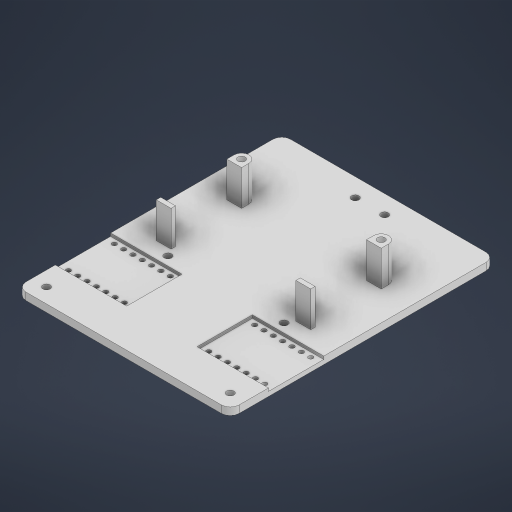
# Autodesk Inventor part: chasis
Saved by Autodesk Inventor 2023 (Build 270158000, 158)
## iProperties
Created: 2022-08-21
Part Number: chasis
Material: Generic
Document SubType Name: Modeling
Designer: marat
Density: 1 g/cm^3
Appearance: Default
Author: marat
Autodesk Inventor part; units mm, degrees
ref_plane "YZ Plane" through (0, 0, 0) normal (1, 0, 0) x (0, 1, 0)
ref_plane "XZ Plane" through (0, 0, 0) normal (0, 1, 0) x (-1, 0, 0)
ref_plane "XY Plane" through (0, 0, 0) normal (0, 0, 1) x (1, 0, 0)
sketch "Sketch3" plane through (0, 0, 0) normal (0, 1, 0) x (-1, 0, 0)
  line L0 (72.5, 90) -> (-72.5, 90)
  line L1 (-72.5, 90) -> (-72.5, -90)
  line L2 (-72.5, -90) -> (72.5, -90)
  line L3 (72.5, -90) -> (72.5, 90)
  line L4 (72.5, 90) -> (-72.5, -90) construction
  line L5 (-72.5, 90) -> (72.5, -90) construction
  point P0 (0, 0)
  dimension "d7" = 145
  dimension "d8" = 180
  constraints: 12 end point, 2 midpoint, 2 parallel, 1 horizontal, 1 perpendicular
  measures "d7" distance of L2.end L1.end
  measures "d8" distance of L1.end L0.end
extrude "Extrusion3" add sketch "Sketch3" along normal blind 5
sketch "Sketch4" plane through (0, 5, 0) normal (0, 1, 0) x (1, 0, 0)
  line L0 (23.935, -64) -> (72.5, -64)
  line L1 (72.5, -64) -> (72.5, -26.408)
  line L2 (72.5, -26.408) -> (23.935, -26.408)
  line L3 (23.935, -26.408) -> (23.935, -64)
  line L4 (23.935, -64) -> (72.5, -26.408) construction
  line L5 (72.5, -64) -> (23.935, -26.408) construction
  line L6 (72.5, -90) -> (72.5, 90) projected
  line L7 (-72.5, -90) -> (72.5, -90) projected
  line L8 (-72.5, -64) -> (-23.935, -64)
  line L9 (-23.935, -64) -> (-23.935, -26.408)
  line L10 (-23.935, -26.408) -> (-72.5, -26.408)
  line L11 (-72.5, -26.408) -> (-72.5, -64)
  line L12 (-72.5, -64) -> (-23.935, -26.408) construction
  line L13 (-23.935, -64) -> (-72.5, -26.408) construction
  line L14 (-72.5, 90) -> (-72.5, -90) projected
  point P0 (0, 0)
  point P1 (48.2175, -45.204)
  point P2 (-48.2175, -45.204)
  dimension "d11" = 48.565
  dimension "d12" = 37.592
  dimension "d13" = 0
  dimension "d14" = 26
  dimension "d20" = 48.565
  dimension "d21" = 37.592
  dimension "d22" = 0
  dimension "d23" = 26
  constraints: 24 end point, 4 midpoint, 4 parallel, 2 horizontal, 2 perpendicular
  measures "d11" distance of L2.end L1.end
  measures "d12" distance of L1.end L0.end
  measures "d13" distance between parallel lines of L6 L1
  measures "d14" distance between parallel lines of L7 L0
  measures "d20" distance of L10.end L9.end
  measures "d21" distance of L9.end L8.end
  measures "d22" distance between parallel lines of L14 L11
  measures "d23" distance between parallel lines of L7 L8
extrude "Extrusion4" cut sketch "Sketch4" against normal blind 2
sketch "Sketch5" plane through (0, 3, 0) normal (0, 1, 0) x (1, 0, 0)
  circle A0 centre (66.797, -60.825) radius 1.588
  line L0 (72.5, -26.408) -> (72.5, -64)
  line L1 (72.5, -64) -> (23.935, -64)
  circle A1 centre (60.447, -60.825) radius 1.588
  circle A2 centre (54.097, -60.825) radius 1.588
  circle A3 centre (47.747, -60.825) radius 1.588
  circle A4 centre (41.397, -60.825) radius 1.588
  circle A5 centre (35.047, -60.825) radius 1.588
  circle A6 centre (28.697, -60.825) radius 1.588
  circle A7 centre (66.797, -29.583) radius 1.588
  circle A8 centre (60.447, -29.583) radius 1.588
  circle A9 centre (54.097, -29.583) radius 1.588
  circle A10 centre (47.747, -29.583) radius 1.588
  circle A11 centre (41.397, -29.583) radius 1.588
  circle A12 centre (35.047, -29.583) radius 1.588
  circle A13 centre (28.697, -29.583) radius 1.588
  circle A14 centre (-66.797, -60.825) radius 1.588
  line L2 (-23.935, -64) -> (-72.5, -64) projected
  line L3 (-72.5, -64) -> (-72.5, -26.408) projected
  circle A15 centre (-60.447, -60.825) radius 1.588
  circle A16 centre (-54.097, -60.825) radius 1.588
  circle A17 centre (-47.747, -60.825) radius 1.588
  circle A18 centre (-41.397, -60.825) radius 1.588
  circle A19 centre (-35.047, -60.825) radius 1.588
  circle A20 centre (-28.697, -60.825) radius 1.588
  circle A21 centre (-66.797, -29.583) radius 1.588
  circle A22 centre (-60.447, -29.583) radius 1.588
  circle A23 centre (-54.097, -29.583) radius 1.588
  circle A24 centre (-47.747, -29.583) radius 1.588
  circle A25 centre (-41.397, -29.583) radius 1.588
  circle A26 centre (-35.047, -29.583) radius 1.588
  circle A27 centre (-28.697, -29.583) radius 1.588
  point P0 (0, 0)
  dimension "d24" = 3.176
  dimension "d25" = 5.703
  dimension "d26" = 3.175
  dimension "d30" = 6.35
  dimension "d33" = 31.242
  dimension "d36" = 3.176
  dimension "d37" = 3.175
  dimension "d38" = 5.703
  dimension "d41" = 6.35
  dimension "d44" = 31.242
  constraints: 28 centre point, 4 end point, 2 horizontal, 2 vertical, 52 other
  measures "d24" diameter of A0
  measures "d25" distance from line of L0 A0.centre
  measures "d26" distance from line of L1 A0.centre
  measures "d30" distance of A0.centre A1.centre
  measures "d33" distance of A0.centre A7.centre
  measures "d36" diameter of A14
  measures "d37" distance from line of L2 A14.centre
  measures "d38" distance from line of L3 A14.centre
  measures "d41" distance of A14.centre A15.centre
  measures "d44" distance of A14.centre A21.centre
extrude "Extrusion5" cut sketch "Sketch5" against normal through all
sketch "Sketch6" plane through (0, 5, 0) normal (0, 1, 0) x (1, 0, 0)
  line L0 (42.5, 32.6926) -> (52.5, 32.6926)
  line L1 (52.5, 32.6926) -> (52.5, 37.6926)
  line L2 (52.5, 37.6926) -> (42.5, 37.6926)
  line L3 (42.5, 37.6926) -> (42.5, 32.6926)
  line L4 (42.5, 32.6926) -> (52.5, 37.6926) construction
  line L5 (52.5, 32.6926) -> (42.5, 37.6926) construction
  line L6 (72.5, -26.408) -> (72.5, 90) projected
  line L7 (-52.5, 32.6926) -> (-42.5, 32.6926)
  line L8 (-42.5, 32.6926) -> (-42.5, 37.6926)
  line L9 (-42.5, 37.6926) -> (-52.5, 37.6926)
  line L10 (-52.5, 37.6926) -> (-52.5, 32.6926)
  line L11 (-52.5, 32.6926) -> (-42.5, 37.6926) construction
  line L12 (-42.5, 32.6926) -> (-52.5, 37.6926) construction
  line L13 (-72.5, 90) -> (-72.5, -26.408) projected
  line L14 (-52.5, -15.3074) -> (-42.5, -15.3074)
  line L15 (-42.5, -15.3074) -> (-42.5, -12.3074)
  line L16 (-42.5, -12.3074) -> (-52.5, -12.3074)
  line L17 (-52.5, -12.3074) -> (-52.5, -15.3074)
  line L18 (-52.5, -15.3074) -> (-42.5, -12.3074) construction
  line L19 (-42.5, -15.3074) -> (-52.5, -12.3074) construction
  line L20 (42.5, -15.3074) -> (52.5, -15.3074)
  line L21 (52.5, -15.3074) -> (52.5, -12.3074)
  line L22 (52.5, -12.3074) -> (42.5, -12.3074)
  line L23 (42.5, -12.3074) -> (42.5, -15.3074)
  line L24 (42.5, -15.3074) -> (52.5, -12.3074) construction
  line L25 (52.5, -15.3074) -> (42.5, -12.3074) construction
  arc A0 (-42.5, 37.6926) -> (-52.5, 37.6926) centre (-47.5, 37.6926) ccw
  arc A1 (52.5, 37.6926) -> (42.5, 37.6926) centre (47.5, 37.6926) ccw
  line L26 (-72.5, -26.408) -> (-23.935, -26.408) projected
  line L27 (23.935, -26.408) -> (72.5, -26.408) projected
  point P0 (0, 0)
  point P1 (47.5, 35.1926)
  point P2 (-47.5, 35.1926)
  point P3 (-47.5, -13.8074)
  point P4 (47.5, -13.8074)
  dimension "d49" = 10
  dimension "d50" = 5
  dimension "d51" = 20
  dimension "d52" = 10
  dimension "d53" = 5
  dimension "d54" = 20
  dimension "d57" = 10
  dimension "d58" = 3
  dimension "d59" = 10
  dimension "d60" = 3
  dimension "d61" = 45
  dimension "d84" = 11.1006
  dimension "d85" = 11.1006
  constraints: 48 end point, 10 midpoint, 8 parallel, 4 horizontal, 4 perpendicular, 4 point on circle, 3 collinear, 2 centre point
  measures "d49" distance of L2.end L1.end
  measures "d50" distance of L1.end L0.end
  measures "d51" distance between parallel lines of L6 L1
  measures "d52" distance of L9.end L8.end
  measures "d53" distance of L8.end L7.end
  measures "d54" distance between parallel lines of L10 L13
  measures "d57" distance of L16.end L15.end
  measures "d58" distance of L15.end L15.start
  measures "d59" distance of L22.end L21.end
  measures "d60" distance of L21.end L21.start
  measures "d61" distance between parallel lines of L7 L16
  measures "d84" distance between parallel lines of L14 L26
  measures "d85" distance between parallel lines of L20 L27
extrude "Extrusion6" add sketch "Sketch6" along normal blind 24
sketch "Sketch7" plane through (0, 5, 0) normal (0, 1, 0) x (1, 0, 0)
  circle A0 centre (62.5, -80) radius 2.5
  line L0 (72.5, -90) -> (72.5, -64) projected
  line L1 (-72.5, -90) -> (72.5, -90) projected
  circle A1 centre (-62.5, -80) radius 2.5
  line L2 (-72.5, -64) -> (-72.5, -90) projected
  circle A2 centre (-39.5, -20.408) radius 2.5
  line L3 (-42.5, -15.3074) -> (-42.5, -12.3074) projected
  line L4 (-72.5, -26.408) -> (-23.935, -26.408) projected
  circle A3 centre (39.5, -20.408) radius 2.5
  line L5 (42.5, -12.3074) -> (42.5, -15.3074) projected
  line L6 (23.935, -26.408) -> (72.5, -26.408) projected
  line L7 (52.5, 35.6926) -> (42.5, 35.6926) projected
  circle A4 centre (39.5, -20.408) radius 4
  circle A5 centre (-39.5, -20.408) radius 4
  circle A6 centre (-62.5, -80) radius 4
  circle A7 centre (62.5, -80) radius 4
  circle A8 centre (-10, 77.5) radius 2.5
  line L8 (72.5, 90) -> (-72.5, 90) projected
  circle A9 centre (10, 77.5) radius 2.5
  point P0 (0, 0)
  point P1 (52.5, 37.6926)
  point P2 (42.5, 37.6926)
  point P3 (0, 90)
  point P4 (0, 90)
  dimension "d63" = 5
  dimension "d64" = 10
  dimension "d65" = 10
  dimension "d66" = 5
  dimension "d67" = 10
  dimension "d68" = 10
  dimension "d69" = 5
  dimension "d70" = 3
  dimension "d71" = 6
  dimension "d72" = 5
  dimension "d73" = 3
  dimension "d74" = 6
  dimension "d80" = 1.5
  dimension "d81" = 1.5
  dimension "d82" = 1.5
  dimension "d83" = 1.5
  dimension "d90" = 5
  dimension "d91" = 12.5
  dimension "d92" = 10
  dimension "d93" = 5
  dimension "d94" = 10
  constraints: 10 centre point, 2 midpoint
  measures "d63" diameter of A0
  measures "d64" distance from line of L0 A0.centre
  measures "d65" distance from line of L1 A0.centre
  measures "d66" diameter of A1
  measures "d67" distance from line of L2 A1.centre
  measures "d68" distance from line of L1 A1.centre
  measures "d69" diameter of A2
  measures "d70" distance from line of L3 A2.centre
  measures "d71" distance from line of L4 A2.centre
  measures "d72" diameter of A3
  measures "d73" distance from line of L5 A3.centre
  measures "d74" distance from line of L6 A3.centre
  measures "d80" radial gap between concentric circles of A3 A4
  measures "d81" radial gap between concentric circles of A2 A5
  measures "d82" radial gap between concentric circles of A1 A6
  measures "d83" radial gap between concentric circles of A0 A7
  measures "d90" diameter of A8
  measures "d91" distance from line of L8 A8.centre
  measures "d92" horizontal distance of point (0, 90) A8.centre
  measures "d93" diameter of A9
  measures "d94" horizontal distance of A9.centre point (0, 90)
extrude "Extrusion7" cut sketch "Sketch7" against normal through all contours A0 | A1 | A2 | A3 | A8 | A9
sketch "Sketch8" plane through (0, 29, 0) normal (0, 1, 0) x (1, 0, 0)
  line L0 (-42.5, 32.6926) -> (-52.5, 32.6926) projected
  line L1 (-47.5, 32.6926) -> (-47.5, 42.6926)
  arc A0 (-42.5, 37.6926) -> (-52.5, 37.6926) centre (-47.5, 37.6926) ccw projected
  line L2 (42.5, 32.6926) -> (52.5, 32.6926) projected
  line L3 (47.5, 32.6926) -> (47.5, 42.6926)
  arc A1 (52.5, 37.6926) -> (42.5, 37.6926) centre (47.5, 37.6926) ccw projected
  circle A2 centre (47.5, 37.6926) radius 2.5
  circle A3 centre (-47.5, 37.6926) radius 2.5
  point P0 (0, 0)
  dimension "d86" = 5
  dimension "d87" = 5
  constraints: 4 end point, 2 centre point, 2 coincident, 2 midpoint, 2 point on circle, 1 parallel, 1 vertical
  measures "d86" diameter of A2
  measures "d87" diameter of A3
extrude "Extrusion8" cut sketch "Sketch8" against normal blind 10
fillet "Fillet1" radius 6 4 edges at (72.5, 2.5, 90) (-72.5, 2.5, 90) (-72.5, 2.5, -90) (72.5, 2.5, -90)
body "Solid2"
